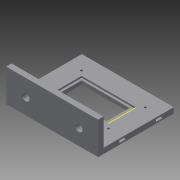
# Autodesk Inventor part: SampleBase
Saved by Autodesk Inventor 2015 (Build 190159000, 159)
## iProperties
Created: 2014-06-06
Part Number: SampleBase
Material: Generic
Document SubType Name: Modeling
Designer: miles90
Density: 1 g/cm^3
Appearance: Default
Author: miles90
Autodesk Inventor part; units mm, degrees
ref_plane "YZ Plane" through (0, 0, 0) normal (1, 0, 0) x (0, 1, 0)
ref_plane "XZ Plane" through (0, 0, 0) normal (0, 1, 0) x (-1, 0, 0)
ref_plane "XY Plane" through (0, 0, 0) normal (0, 0, 1) x (1, 0, 0)
sketch "Sketch1" plane through (0, 0, 0) normal (0, 1, 0) x (-1, 0, 0)
  line L0 (52.3087, -21.6726) -> (-32.6913, -21.6726)
  line L1 (-32.6913, -21.6726) -> (-32.6913, 48.3274)
  line L2 (-32.6913, 48.3274) -> (52.3087, 48.3274)
  line L3 (52.3087, 48.3274) -> (52.3087, -21.6726)
  dimension "d4" = 70
  dimension "d5" = 85
  constraints: 8 end point, 2 parallel, 1 horizontal, 1 perpendicular
  measures "d4" distance of L2.end L0.start
  measures "d5" distance of L0.start L0.end
extrude "Extrusion1" add sketch "Sketch1" along normal blind 30
sketch "Sketch2" plane through (0, 30, 0) normal (0, 1, 0) x (1, 0, 0)
  line L0 (32.6913, 21.6726) -> (-52.3087, 21.6726) projected
  line L1 (-52.3087, 21.6726) -> (-52.3087, -48.3274) projected
  line L2 (-52.3087, -48.3274) -> (32.6913, -48.3274) projected
  line L3 (32.6913, -48.3274) -> (32.6913, 21.6726) projected
  line L4 (-52.3087, 21.6726) -> (32.6913, 21.6726)
  line L5 (32.6913, 21.6726) -> (32.6913, -43.3274)
  line L6 (32.6913, -43.3274) -> (-52.3087, -43.3274)
  line L7 (-52.3087, -43.3274) -> (-52.3087, 21.6726)
  point P0 (0, 0)
  dimension "d8" = 0
  dimension "d9" = 0
  dimension "d10" = 5
  constraints: 8 end point, 1 collinear, 1 parallel, 1 perpendicular
  measures "d8" distance between parallel lines of L1 L7
  measures "d9" distance between parallel lines of L5 L3
  measures "d10" distance between parallel lines of L6 L2
extrude "Extrusion2" cut sketch "Sketch2" against normal blind 25 contours L3 L6 L1 L0
sketch "Sketch3" plane through (0, 5, 0) normal (0, 1, 0) x (1, 0, 0)
  line L0 (-52.3087, -43.3274) -> (-52.3087, 21.6726) projected
  line L1 (32.6913, -43.3274) -> (-52.3087, -43.3274) projected
  line L2 (32.6913, 21.6726) -> (32.6913, -43.3274) projected
  line L3 (-34.9087, 4.0726) -> (15.2913, 4.0726)
  line L4 (15.2913, 4.0726) -> (15.2913, -21.4274)
  line L5 (15.2913, -21.4274) -> (-34.9087, -21.4274)
  line L6 (-34.9087, -21.4274) -> (-34.9087, 4.0726)
  line L7 (-52.3087, 21.6726) -> (32.6913, 21.6726)
  line L8 (-52.3087, -48.3274) -> (-52.3087, 21.6726) projected
  line L9 (-9.8087, -43.3274) -> (-9.8087, 21.6726) construction
  circle A0 centre (-39.3087, -25.6774) radius 1
  circle A1 centre (-39.3087, 8.3226) radius 1
  circle A2 centre (19.6913, 8.3226) radius 1
  circle A3 centre (19.6913, -25.6774) radius 1
  line L10 (-34.9087, -8.6774) -> (15.2913, -8.6774) construction
  point P0 (0, 0)
  dimension "d14" = 17.4
  dimension "d15" = 17.4
  dimension "d17" = 21.9
  dimension "d106" = 25.5
  dimension "d107" = 2
  dimension "d110" = 34
  dimension "d111" = 59
  constraints: 14 end point, 4 centre point, 4 midpoint, 4 perpendicular, 3 equal radius, 3 symmetric about line, 2 parallel, 1 horizontal, 2 other
  measures "d14" distance between parallel lines of L2 L4
  measures "d15" distance between parallel lines of L0 L6
  measures "d17" distance between parallel lines of L5 L1
  measures "d106" distance between parallel lines of L3 L5
  measures "d107" diameter of A0
  measures "d110" distance of A1.centre A0.centre
  measures "d111" distance of A0.centre A3.centre
extrude "Extrusion3" cut sketch "Sketch3" against normal blind 1.5 contours L3 L4 L5 L6 | A0 | A1 | A2 | A3
sketch "Sketch4" plane through (0, 3.5, 0) normal (0, 1, 0) x (1, 0, 0)
  line L0 (-34.9087, 4.0726) -> (15.2913, 4.0726) projected
  line L1 (-34.9087, -21.4274) -> (-34.9087, 4.0726) projected
  line L2 (15.2913, -21.4274) -> (-34.9087, -21.4274) projected
  line L3 (15.2913, 4.0726) -> (15.2913, -21.4274) projected
  line L4 (-32.9087, 2.0726) -> (11.2913, 2.0726)
  line L5 (11.2913, 2.0726) -> (11.2913, -19.4274)
  line L6 (11.2913, -19.4274) -> (-32.9087, -19.4274)
  line L7 (-32.9087, -19.4274) -> (-32.9087, 2.0726)
  point P0 (0, 0)
  dimension "d20" = 2
  dimension "d21" = 2
  dimension "d22" = 2
  dimension "d23" = 4
  constraints: 8 end point, 2 parallel, 1 horizontal, 1 perpendicular
  measures "d20" distance between parallel lines of L1 L7
  measures "d21" distance between parallel lines of L0 L4
  measures "d22" distance between parallel lines of L2 L6
  measures "d23" distance between parallel lines of L3 L5
extrude "Extrusion4" cut sketch "Sketch4" against normal blind 1 contours L4 L5 L6 L7
sketch "Sketch10" plane through (32.6913, 5, 43.3274) normal (0, 0, -1) x (-1, 0, 0)
  line L0 (85, 25) -> (85, 0) projected
  line L1 (0, 25) -> (85, 25) projected
  circle A0 centre (18, 9.75) radius 3.5
  circle A1 centre (67, 9.75) radius 3.5
  point P0 (32.6913, -5)
  dimension "d53" = 15.25
  dimension "d55" = 15.25
  dimension "d58" = 7
  dimension "d59" = 7
  dimension "d70" = 49
  dimension "d71" = 18
  constraints: 2 centre point
  measures "d53" distance from line of L1 A1.centre
  measures "d55" distance from line of L1 A0.centre
  measures "d58" diameter of A0
  measures "d59" diameter of A1
  measures "d70" distance of A1.centre A0.centre
  measures "d71" distance from line of L0 A1.centre
extrude "Extrusion9" cut sketch "Sketch10" against normal blind 5
sketch "Sketch16" plane through (15.2913, 5, -4.0726) normal (-1, 0, 0) x (0, 0, 1)
  line L0 (0, 0) -> (25.5, 0) projected
  line L1 (0, 0) -> (0, -1.5) projected
  line L2 (0, -1.5) -> (25.5, -1.5) projected
  line L3 (25.5, 0) -> (25.5, -1.5) projected
  point P0 (4.0726, -5)
sketch "Sketch17" plane through (0, 2.5, 0) normal (0, 1, 0) x (1, 0, 0)
  line L0 (-32.9087, 2.0726) -> (11.2913, 2.0726) projected
  line L1 (-32.9087, -19.4274) -> (-32.9087, 2.0726) projected
  line L2 (11.2913, -19.4274) -> (-32.9087, -19.4274) projected
  line L3 (11.2913, 2.0726) -> (11.2913, -19.4274) projected
  line L4 (-32.9087, 2.0726) -> (11.2913, 2.0726)
  line L5 (11.2913, 2.0726) -> (11.2913, -19.4274)
  line L6 (11.2913, -19.4274) -> (-32.9087, -19.4274)
  line L7 (-32.9087, -19.4274) -> (-32.9087, 2.0726)
  point P0 (0, 0)
  dimension "d93" = 0
  dimension "d94" = 0
  dimension "d95" = 0
  dimension "d96" = 0
  constraints: 8 end point, 2 parallel, 1 horizontal, 1 perpendicular
  measures "d93" distance between parallel lines of L0 L4
  measures "d94" distance between parallel lines of L3 L5
  measures "d95" distance between parallel lines of L1 L7
  measures "d96" distance between parallel lines of L2 L6
extrude "Extrusion14" cut sketch "Sketch17" along normal through all both and the other way through all
sketch "Sketch20" plane through (32.6913, 0, 48.3274) normal (1, 0, 0) x (0, 0, -1)
  line L0 (19.65, 3.5) -> (25.65, 3.5)
  line L1 (25.65, 3.5) -> (25.65, 1.5)
  line L2 (25.65, 1.5) -> (19.65, 1.5)
  line L3 (19.65, 1.5) -> (19.65, 3.5)
  line L4 (53.65, 3.5) -> (59.65, 3.5)
  line L5 (59.65, 3.5) -> (59.65, 1.5)
  line L6 (59.65, 1.5) -> (53.65, 1.5)
  line L7 (53.65, 1.5) -> (53.65, 3.5)
  line L8 (21.65, 3.5) -> (23.65, 3.5) construction
  line L9 (55.65, 3.5) -> (57.65, 3.5) construction
  point P0 (48.3274, 0)
  dimension "d113" = 2
  dimension "d119" = 2
  dimension "d124" = 6
  dimension "d125" = 6
  dimension "d128" = 2
  dimension "d129" = 2
  constraints: 16 end point, 4 parallel, 2 collinear, 1 horizontal, 1 perpendicular
  measures "d113" distance of L0.end L1.end
  measures "d119" distance of L4.end L5.end
  measures "d124" distance between parallel lines of L5 L7
  measures "d125" distance between parallel lines of L1 L3
  measures "d128" distance from line of L7 L9.start
  measures "d129" distance from line of L8.start L3
extrude "Extrusion16" cut sketch "Sketch20" against normal blind 16
sketch "Sketch21" plane through (-52.3087, 0, -21.6726) normal (-1, 0, 0) x (0, 0, 1)
  line L0 (17.6, 3.5) -> (43.1, 3.5) projected
  line L1 (10.35, 1.5) -> (16.35, 1.5)
  line L2 (16.35, 1.5) -> (16.35, 3.5)
  line L3 (16.35, 3.5) -> (10.35, 3.5)
  line L4 (10.35, 3.5) -> (10.35, 1.5)
  line L5 (44.35, 1.5) -> (50.35, 1.5)
  line L6 (50.35, 1.5) -> (50.35, 3.5)
  line L7 (50.35, 3.5) -> (44.35, 3.5)
  line L8 (44.35, 3.5) -> (44.35, 1.5)
  line L9 (10.35, 3.5) -> (10.35, 1.5) projected
  line L10 (10.35, 1.5) -> (16.35, 1.5) projected
  line L11 (16.35, 1.5) -> (16.35, 3.5) projected
  line L12 (50.35, 1.5) -> (50.35, 3.5) projected
  line L13 (44.35, 1.5) -> (50.35, 1.5) projected
  line L14 (44.35, 3.5) -> (44.35, 1.5) projected
  point P0 (21.6726, 0)
  constraints: 16 end point, 8 collinear, 4 parallel, 2 horizontal, 2 perpendicular, 1 point on line
extrude "Extrusion17" cut sketch "Sketch21" against normal blind 16
body "Solid1"
